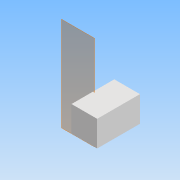
# Autodesk Inventor part: 車體上做
Saved by Autodesk Inventor 2021 (Build 250183000, 183)
## iProperties
Created: 2025-12-12
Part Number: 車體上做
Material: 一般
Document SubType Name: Modeling
Designer: User
Density: 1 g/cm^3
Appearance: 預設
Author: User
Autodesk Inventor part; units mm, degrees
ref_plane "YZ Plane" through (0, 0, 0) normal (1, 0, 0) x (0, 1, 0)
ref_plane "XZ Plane" through (0, 0, 0) normal (0, 1, 0) x (-1, 0, 0)
ref_plane "XY Plane" through (0, 0, 0) normal (0, 0, 1) x (1, 0, 0)
ref_plane "工作平面1" through (0, 0, 0) normal (0, 0, 1) x (1, 0, 0)
sketch "草圖1" plane through (0, 0, 0) normal (0, 0, 1) x (1, 0, 0)
  line L0 (-247.7976, 597.9344) -> (-247.7976, -597.9344)
  line L1 (-247.7976, -597.9344) -> (183.7246, -900)
  line L2 (183.7246, -900) -> (252.2024, -900)
  line L3 (252.2024, -900) -> (252.2024, 597.9344)
  line L4 (252.2024, 597.9344) -> (-247.7976, 597.9344)
  circle A0 centre (32.2024, 865) radius 22.5
  line L5 (212.2024, 785) -> (352.2024, 785)
  line L6 (352.2024, 785) -> (352.2024, -1000)
  line L7 (352.2024, -1000) -> (152.2024, -1000)
  line L8 (152.2024, -1000) -> (-347.7976, -650)
  line L9 (-347.7976, -650) -> (-347.7976, 650)
  line L10 (-347.7976, 650) -> (-154.9405, 785)
  line L11 (-154.9405, 785) -> (212.2024, 785)
  circle A1 centre (212.2024, 875) radius 90
  line L12 (-247.7976, 597.9344) -> (-247.7976, -597.9344)
  line L13 (-247.7976, -597.9344) -> (183.7246, -900)
  line L14 (183.7246, -900) -> (252.2024, -900)
  line L15 (252.2024, -900) -> (252.2024, 597.9344)
  line L16 (252.2024, 597.9344) -> (-247.7976, 597.9344)
  circle A2 centre (32.2024, 865) radius 22.5
  line L17 (212.2024, 785) -> (352.2024, 785)
  line L18 (352.2024, 785) -> (352.2024, -1000)
  line L19 (352.2024, -1000) -> (152.2024, -1000)
  line L20 (152.2024, -1000) -> (-347.7976, -650)
  line L21 (-347.7976, -650) -> (-347.7976, 650)
  line L22 (-347.7976, 650) -> (-154.9405, 785)
  line L23 (-154.9405, 785) -> (212.2024, 785)
  circle A3 centre (212.2024, 875) radius 90
  circle A4 centre (-197.7976, -571.9017) radius 50 projected
  circle A5 centre (-197.7976, 547.9344) radius 50 projected
  line L24 (352.2024, -1000) -> (352.2024, 1000) projected
  line L25 (-347.7976, -650) -> (-347.7976, 650) projected
  line L26 (-347.7976, 650) -> (152.2024, 1000) projected
  line L27 (152.2024, 1000) -> (352.2024, 1000) projected
  line L28 (352.2024, 0) -> (952.2024, 0)
  line L29 (952.2024, 0) -> (952.2024, -600)
  line L30 (952.2024, -600) -> (352.2024, -600)
  line L31 (352.2024, -600) -> (352.2024, 0)
  line L32 (352.2024, -1000) -> (152.2024, -1000) projected
  line L33 (152.2024, -1000) -> (-347.7976, -650) projected
  point P0 (0, 0)
  dimension "d0" = 600
  dimension "d1" = 600
  constraints: 56 end point, 11 horizontal, 8 vertical, 2 centre point, 2 parallel, 2 vertical alignment, 1 midpoint, 1 perpendicular, 26 other
  measures "d0" distance of L29.end L30.end
  measures "d1" distance between parallel lines of L30 L28
extrude "擠出1" add sketch "草圖1" along normal mid plane 1000 contours L28 L29 L30 L6
